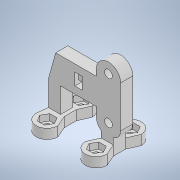
# Autodesk Inventor part: Крепление двигателя
Saved by Autodesk Inventor 2020 (Build 240168000, 168)
## iProperties
Created: 2021-05-24
Part Number: Крепление двигателя
Material: Типовые
Document SubType Name: Modeling
Designer: Антон
Density: 1 g/cm^3
Appearance: По умолчанию
Author: Антон
Autodesk Inventor part; units mm, degrees
ref_plane "YZ Plane" through (0, 0, 0) normal (1, 0, 0) x (0, 1, 0)
ref_plane "XZ Plane" through (0, 0, 0) normal (0, 1, 0) x (-1, 0, 0)
ref_plane "XY Plane" through (0, 0, 0) normal (0, 0, 1) x (1, 0, 0)
sketch "Эскиз1" plane through (0, 0, 0) normal (0, 0, 1) x (1, 0, 0)
  line L0 (0, 0) -> (26.75, 0)
  line L1 (26.75, 0) -> (26.75, 26)
  line L2 (26.75, 26) -> (0, 26)
  line L3 (0, 26) -> (0, 0)
  line L4 (0, 0) -> (16.75, 0)
  line L5 (16.75, 0) -> (16.75, 7.6)
  line L6 (16.75, 7.6) -> (0, 7.6)
  line L7 (0, 7.6) -> (0, 0)
  line L8 (0, 26) -> (16.75, 26)
  line L9 (16.75, 26) -> (16.75, 18.4)
  line L10 (16.75, 18.4) -> (0, 18.4)
  line L11 (0, 18.4) -> (0, 26)
  point P0 (0, 7.6)
  dimension "d0" = 26.75
  dimension "d1" = 26
  dimension "d14" = 16.75
  dimension "d15" = 7.6
  constraints: 24 end point, 6 parallel, 3 horizontal, 3 perpendicular, 2 equal length
  measures "d0" distance of L2.end L1.end
  measures "d1" distance of L1.end L0.end
  measures "d14" distance of L6.end L5.end
  measures "d15" distance of L5.end L4.end
extrude "Выдавливание1" add sketch "Эскиз1" along normal blind 5 contours L5 L6 L3 L10 L9 L2 L1 L0
sketch "Эскиз2" plane through (0, 0, 5) normal (0, 0, 1) x (1, 0, 0)
  line L0 (26.75, 0) -> (26.75, 26) projected
  line L1 (26.75, 13) -> (21.75, 13)
  line L2 (21.75, 13) -> (21.75, 21.75)
  line L3 (21.75, 13) -> (21.75, 4.25)
  point P0 (0, 0)
  dimension "d4" = 5
  dimension "d6" = 17.5
  constraints: 6 end point, 1 collinear, 1 horizontal, 1 midpoint, 1 perpendicular, 1 vertical
  measures "d4" distance of L1.start L1.end
  measures "d6" distance of L3.end L2.end
hole "Отверстие1" at (21.75, 21.75, 5) at (21.75, 4.25, 5) direction (0, 0, -1) diameter 3.2 end through all
sketch "Эскиз4" plane through (0, 0, 0) normal (0, 0, -1) x (-1, 0, 0)
  line L0 (-23.75, 0) -> (-18.75, 0)
  line L1 (-18.75, 0) -> (-18.75, -6.62)
  line L2 (-18.75, -6.62) -> (-23.75, -6.62)
  line L3 (-23.75, -6.62) -> (-23.75, 0)
  line L4 (3, 7.6) -> (-2, 7.6)
  line L5 (-2, 7.6) -> (-2, -6.62)
  line L6 (-2, -6.62) -> (3, -6.62)
  line L7 (3, -6.62) -> (3, 7.6)
  line L8 (-16.75, 0) -> (-26.75, 0) projected
  line L9 (-26.75, 0) -> (-26.75, 26) projected
  line L10 (0, 7.6) -> (-16.75, 7.6) projected
  line L11 (0, 18.4) -> (0, 7.6) projected
  point P0 (0, 0)
  dimension "d20" = 5
  dimension "d21" = 6.62
  dimension "d22" = 5
  dimension "d82" = 3
  dimension "d83" = 3
  constraints: 16 end point, 4 parallel, 3 collinear, 2 horizontal, 2 perpendicular
  measures "d20" distance of L1.end L2.end
  measures "d21" distance of L0.end L1.end
  measures "d22" distance of L6.end L5.end
  measures "d82" distance between parallel lines of L3 L9
  measures "d83" distance between parallel lines of L11 L7
extrude "Выдавливание3" add sketch "Эскиз4" against normal up to surface (5 mm away)
sketch "Эскиз5" plane through (18.75, -6.62, 0) normal (0, -1, 0) x (1, 0, 0)
  line L0 (6.9685, 0) -> (-1.9685, 0)
  line L1 (-1.9685, 0) -> (-1.9685, -9.008)
  line L2 (-1.9685, -9.008) -> (6.9685, -9.008)
  line L3 (6.9685, -9.008) -> (6.9685, 0)
  line L4 (5, 0) -> (0, 0) projected
  line L5 (-13.2815, 0) -> (-22.2185, 0)
  line L6 (-22.2185, 0) -> (-22.2185, -9.008)
  line L7 (-22.2185, -9.008) -> (-13.2815, -9.008)
  line L8 (-13.2815, -9.008) -> (-13.2815, 0)
  line L9 (-16.75, 0) -> (-18.75, 0) projected
  line L10 (-1.9685, -4.504) -> (6.9685, -4.504)
  line L11 (-13.2815, -4.504) -> (-22.2185, -4.504)
  circle A0 centre (-17.75, -4.504) radius 1.6
  circle A1 centre (2.5, -4.504) radius 1.6
  point P0 (2.5, 0)
  point P1 (-17.75, 0)
  dimension "d25" = 8.937
  dimension "d26" = 9.008
  dimension "d27" = 8.937
  dimension "d28" = 9.008
  dimension "d64" = 3.2
  dimension "d65" = 3.2
  constraints: 20 end point, 10 midpoint, 4 parallel, 2 centre point, 2 horizontal, 2 perpendicular
  measures "d25" distance of L2.end L1.end
  measures "d26" distance of L1.end L0.end
  measures "d27" distance of L7.end L6.end
  measures "d28" distance of L6.end L5.end
  measures "d64" diameter of A0
  measures "d65" diameter of A1
extrude "Выдавливание4" add sketch "Эскиз5" against normal blind 4 contours L3 L10 A1 L1 L0 | L3 L2 L1 L10 A1 | L8 L11 A0 L6 L5 | L8 L7 L6 L11 A0
sketch "Эскиз12" plane through (18.75, -2.62, 0) normal (0, 1, 0) x (1, 0, 0)
  circle A0 centre (-17.75, 4.504) radius 1.6 projected
  circle A1 centre (2.5, 4.504) radius 1.6 projected
  line L0 (-16.2489, 7.104) -> (-14.7478, 4.504)
  line L1 (-14.7478, 4.504) -> (-16.2489, 1.904)
  line L2 (-16.2489, 1.904) -> (-19.2511, 1.904)
  line L3 (-19.2511, 1.904) -> (-20.7522, 4.504)
  line L4 (-20.7522, 4.504) -> (-19.2511, 7.104)
  line L5 (-19.2511, 7.104) -> (-16.2489, 7.104)
  line L6 (4.0011, 7.104) -> (5.5022, 4.504)
  line L7 (5.5022, 4.504) -> (4.0011, 1.904)
  line L8 (4.0011, 1.904) -> (0.9989, 1.904)
  line L9 (0.9989, 1.904) -> (-0.5022, 4.504)
  line L10 (-0.5022, 4.504) -> (0.9989, 7.104)
  line L11 (0.9989, 7.104) -> (4.0011, 7.104)
  line L12 (-13.2815, 9.008) -> (-22.2185, 9.008) projected
  line L13 (6.9685, 9.008) -> (-1.9685, 9.008) projected
  point P0 (-18.75, 0)
  dimension "d66" = 5.2
  constraints: 24 end point, 2 coincident, 2 parallel, 1 collinear, 26 other
  measures "d66" distance between parallel lines of L5 L2
extrude "Выдавливание10" cut sketch "Эскиз12" against normal blind 2.6 contours A0 | A1 | L0 L1 L2 L3 L4 L5 | L6 L7 L8 L9 L10 L11
fillet "Сопряжение3" radius 4.4685 4 edges at (5.4685, -4.62, -9.008) (-3.4685, -4.62, -9.008) (16.7815, -4.62, -9.008) (25.7185, -4.62, -9.008)
chamfer "Фаска1" distance 4.53 distance2 0.468 1 edges at (-3.4685, -4.62, 0) measured on face at (-3.4685, -4.62, -0.5)
chamfer "Фаска2" distance 1.968 distance2 4.53 1 edges at (25.7185, -4.62, 0) measured on face at (25.2185, -4.62, 0)
chamfer "Фаска3" distance 1.968 distance2 4.53 1 edges at (5.4685, -4.62, 0) measured on face at (4.9685, -4.62, 0)
chamfer "Фаска4" distance 1.968 distance2 4.53 1 edges at (16.7815, -4.62, 0) measured on face at (17.2815, -4.62, 0)
ref_plane "РабПлоскость1" through (0, 0, 2.5) normal (0, 0, -1) x (-1, 0, 0)
mirror "Зеркальное отражение1" about plane through (0, 0, 2.5) normal (0, 0, -1) of "Выдавливание4", "Выдавливание10", "Фаска2", "Фаска4", "Фаска3", "Фаска1", "Сопряжение3"
sketch "Эскиз8" plane through (0, 0, 0) normal (0, 0, -1) x (-1, 0, 0)
  circle A0 centre (-21.75, 21.75) radius 1.6 projected
  line L0 (-23.2511, 19.15) -> (-24.7522, 21.75)
  line L1 (-24.7522, 21.75) -> (-23.2511, 24.35)
  line L2 (-23.2511, 24.35) -> (-20.2489, 24.35)
  line L3 (-20.2489, 24.35) -> (-18.7478, 21.75)
  line L4 (-18.7478, 21.75) -> (-20.2489, 19.15)
  line L5 (-20.2489, 19.15) -> (-23.2511, 19.15)
  circle A1 centre (-21.75, 4.25) radius 1.6 projected
  line L6 (-20.2489, 6.85) -> (-18.7478, 4.25)
  line L7 (-18.7478, 4.25) -> (-20.2489, 1.65)
  line L8 (-20.2489, 1.65) -> (-23.2511, 1.65)
  line L9 (-23.2511, 1.65) -> (-24.7522, 4.25)
  line L10 (-24.7522, 4.25) -> (-23.2511, 6.85)
  line L11 (-23.2511, 6.85) -> (-20.2489, 6.85)
  line L12 (-16.75, 0) -> (-18.75, 0) projected
  line L13 (-26.75, 26) -> (-16.75, 26) projected
  point P0 (0, 0)
  dimension "d42" = 5.2
  constraints: 24 end point, 3 parallel, 2 coincident, 26 other
  measures "d42" distance between parallel lines of L5 L2
sketch "Эскиз9" plane through (0, 0, 0) normal (0, 0, -1) x (-1, 0, 0)
  line L0 (-2, 7.6) -> (-16.75, 7.6) projected
  line L1 (-9.375, 7.6) -> (-9.375, 18.4)
  line L2 (-16.75, 18.4) -> (0, 18.4) projected
  line L3 (-10.875, 10.5) -> (-7.875, 10.5)
  line L4 (-7.875, 10.5) -> (-7.875, 15.5)
  line L5 (-7.875, 15.5) -> (-10.875, 15.5)
  line L6 (-10.875, 15.5) -> (-10.875, 10.5)
  line L7 (-10.875, 10.5) -> (-7.875, 15.5) construction
  line L8 (-7.875, 10.5) -> (-10.875, 15.5) construction
  line L9 (-10.875, 15.5) -> (-7.875, 15.5)
  line L10 (-7.875, 15.5) -> (-7.875, 14)
  line L11 (-7.875, 14) -> (-10.875, 14)
  line L12 (-10.875, 14) -> (-10.875, 15.5)
  line L13 (-10.875, 10.5) -> (-7.875, 10.5)
  line L14 (-7.875, 10.5) -> (-7.875, 12)
  line L15 (-7.875, 12) -> (-10.875, 12)
  line L16 (-10.875, 12) -> (-10.875, 10.5)
  point P0 (0, 0)
  point P1 (-9.375, 13)
  point P2 (-10.875, 12)
  dimension "d45" = 3
  dimension "d46" = 5
  dimension "d47" = 1.5
  dimension "d48" = 1.5
  constraints: 30 end point, 6 parallel, 4 midpoint, 3 horizontal, 3 perpendicular, 3 point on line, 1 vertical
  measures "d45" distance of L5.end L4.end
  measures "d46" distance of L4.end L3.end
  measures "d47" distance of L9.end L10.end
  measures "d48" distance of L14.end L13.end
extrude "Выдавливание7" cut sketch "Эскиз9" against normal through all contours L3 L6 L15 L1 | L1 L15 L4 L3 | L11 L6 L5 L1 | L1 L5 L4 L11
sketch "Эскиз10" plane through (0, 0, 5) normal (0, 0, 1) x (1, 0, 0)
  line L0 (10.875, 12) -> (10.875, 10.5) projected
  line L1 (7.875, 15.5) -> (10.875, 15.5) projected
  line L2 (10.875, 10.5) -> (7.875, 10.5)
  line L3 (7.875, 10.5) -> (7.875, 15.5)
  line L4 (7.875, 15.5) -> (10.875, 15.5)
  line L5 (10.875, 15.5) -> (10.875, 10.5)
  point P0 (0, 0)
  constraints: 8 end point, 2 parallel, 1 horizontal, 1 perpendicular
extrude "Выдавливание8" cut sketch "Эскиз10" against normal blind 1.5
hole "Отверстие3" at (21.75, 21.75, 0) at (21.75, 4.25, 0) direction (0, 0, 1) diameter 3.2 end through all countersink diameter 6 countersink angle 90
fillet "Сопряжение2" radius 5 3 edges at (26.75, 26, 2.5) (16.75, 26, 2.5) (16.75, 0, 2.5)
fillet "Сопряжение2" radius 4 1 edges at (26.75, 0, 2.5)
chamfer "Фаска5" distance 10.8 distance2 3 1 edges at (0, 7.6, 2.5) measured on face at (0, 8.1, 2.5)
sketch "Эскиз13" plane through (3.5005, -6.62, 5) normal (0, 0, -1) x (-1, 0, 0)
  line L0 (0, 0) -> (0, 4) projected
  line L1 (0, 0) -> (1.5005, 0) projected
  line L2 (1.5005, 4) -> (1.5005, 0) projected
  line L3 (1.5005, 4) -> (0, 4) projected
  point P0 (3.5005, 6.62)
extrude "Выдавливание11" add sketch "Эскиз13" along normal up to surface (5 mm away)
